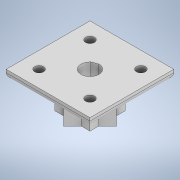
# Autodesk Inventor part: Acople Motor 1
Saved by Autodesk Inventor 2021 (Build 250183000, 183)
## iProperties
Created: 2021-03-15
Part Number: Acople Motor 1
Material: Genérico
Document SubType Name: Modeling
Designer: Joaquín
Density: 1 g/cm^3
Appearance: Valor por defecto
Author: Joaquín
Autodesk Inventor part; units mm, degrees
ref_plane "YZ Plane" through (0, 0, 0) normal (1, 0, 0) x (0, 1, 0)
ref_plane "XZ Plane" through (0, 0, 0) normal (0, 1, 0) x (-1, 0, 0)
ref_plane "XY Plane" through (0, 0, 0) normal (0, 0, 1) x (1, 0, 0)
sketch "Boceto1" plane through (0, 0, 0) normal (0, 1, 0) x (-1, 0, 0)
  line L0 (5.9, 5.9) -> (5.9, 2.95)
  line L1 (-5.9, 5.9) -> (-2.95, 5.9)
  line L2 (5.9, 5.9) -> (2.95, 5.9)
  line L3 (-5.9, -5.9) -> (-5.9, -2.95)
  line L4 (8.85, 0) -> (5.9, 2.95)
  line L5 (8.85, 0) -> (5.9, -2.95)
  line L6 (0, -8.85) -> (-2.95, -5.9)
  line L7 (-8.85, 0) -> (-5.9, -2.95)
  line L8 (-5.9, 2.95) -> (-8.85, 0)
  line L9 (-2.95, 5.9) -> (0, 8.85)
  line L10 (0, 8.85) -> (2.95, 5.9)
  line L11 (2.95, -5.9) -> (0, -8.85)
  line L12 (5.9, -5.9) -> (2.95, -5.9)
  line L13 (-2.95, -5.9) -> (-5.9, -5.9)
  line L14 (5.9, 5.9) -> (5.9, 2.95)
  line L15 (5.9, -2.95) -> (5.9, -5.9)
  line L16 (-5.9, 5.9) -> (-2.95, 5.9)
  line L17 (2.95, 5.9) -> (5.9, 5.9)
  line L18 (-5.9, -5.9) -> (-5.9, -2.95)
  line L19 (-5.9, 2.95) -> (-5.9, 5.9)
  arc A0 (1.9849, -2.2495) -> (0, -3) centre (0, 0) ccw
  line L20 (0, -3) -> (1.9849, -2.2495)
  dimension "d11" = 2.95
  constraints: 42 end point, 9 equal length, 5 perpendicular, 2 horizontal, 2 point on circle, 2 point on line, 1 centre point
  measures "d11" distance of L1.start L1.end
extrude "Extrusión1" add sketch "Boceto1" along normal mid plane 9 contours L0 L4 L5 L15 L12 L11 L6 L13 L3 L7 L8 L19 L1 L9 L10 L2 | L20 A0
sketch "Boceto2" plane through (0, 4.5, 0) normal (0, 1, 0) x (1, 0, 0)
  line L0 (0, -14) -> (-14, -14)
  line L1 (-14, -14) -> (-14, 0)
  line L2 (0, 14) -> (-14, 14)
  line L3 (-14, 14) -> (-14, 0)
  line L4 (0, -14) -> (14, -14)
  line L5 (14, -14) -> (14, 0)
  line L6 (0, 14) -> (14, 14)
  line L7 (14, 14) -> (14, 0)
  line L8 (-14, -14) -> (-14, -9.5)
  circle A0 centre (-9.5, -9.5) radius 1.5
  circle A1 centre (9.5, -9.5) radius 1.5
  circle A2 centre (9.5, 9.5) radius 1.5
  circle A3 centre (-9.5, 9.5) radius 1.5
  point P0 (0, 0)
  dimension "d26" = 4.5
  dimension "d28" = 3
  dimension "d31" = 360
  constraints: 18 end point, 4 centre point, 4 perpendicular, 2 point on line, 1 collinear, 1 horizontal, 9 other
  measures "d26" distance of L0.end L8.end
  measures "d28" diameter of A0
extrude "Extrusión2" add sketch "Boceto2" along normal blind 3 contours L0 L1 L3 L2 L6 L7 L5 L4 | A0 | A1 | A2 | A3
sketch "Boceto5" plane through (0, -4.5, 0) normal (0, -1, 0) x (1, 0, 0)
  arc A0 (0, -3) -> (-1.9849, -2.2495) centre (0, 0) ccw
  line L0 (0, -3) -> (-1.9849, -2.2495)
  dimension "d48" = 6
  constraints: 2 end point, 2 point on circle, 1 centre point, 1 coincident
  measures "d48" diameter of A0
extrude "Extrusión5" cut sketch "Boceto5" along normal mid plane 100
fillet "Empalme1" radius 2 4 edges at (-14, 4.5, 0) (0, 4.5, -14) (14, 4.5, 0) (0, 4.5, 14)
sketch "Boceto6" plane through (0, 7.5, 0) normal (0, 1, 0) x (1, 0, 0)
  line L0 (14, 14) -> (14, -14) projected
  circle A0 centre (8.5, 8.5) radius 1.5
  circle A1 centre (-8.5, 8.5) radius 1.5
  circle A2 centre (-8.5, -8.5) radius 1.5
  circle A3 centre (8.5, -8.5) radius 1.5
  point P0 (0, 0)
  dimension "d68" = 360
  constraints: 4 centre point, 9 other
extrude "Extrusión6" cut sketch "Boceto6" against normal mid plane 100
